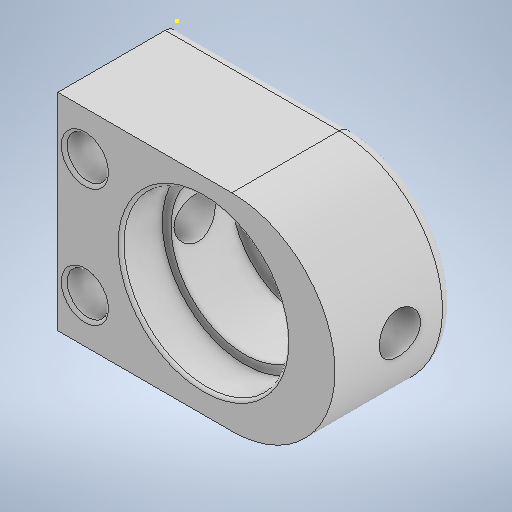
# Autodesk Inventor part: Rodamiento grande
Saved by Autodesk Inventor 2025 (Build 290162000, 162)
## iProperties
Created: 2025-05-21
Part Number: Rodamiento grande
Material: Genérico
Document SubType Name: Modeling
Designer: STEVEN LONDOÑO
Density: 1 g/cm^3
Appearance: Valor por defecto
Author: STEVEN LONDOÑO
Autodesk Inventor part; units mm, degrees
ref_plane "YZ Plane" through (0, 0, 0) normal (1, 0, 0) x (0, 1, 0)
ref_plane "XZ Plane" through (0, 0, 0) normal (0, 1, 0) x (-1, 0, 0)
sketch "Boceto1" plane through (0, 0, 0) normal (0, 0, 1) x (1, 0, 0)
  line L0 (42.7171, -0.3462) -> (13.2171, -0.3462)
  circle A0 centre (37.9098, -17.5) radius 13.97
  line L1 (13.2171, -0.3462) -> (13.2171, -35.3462)
  line L2 (13.2171, -0.3462) -> (13.2171, -35.3462)
  line L3 (13.2171, -35.3462) -> (42.7171, -35.3462)
  arc A1 (42.7171, -35.3462) -> (42.7171, -0.3462) centre (42.7171, -17.8462) ccw
  circle A2 centre (37.9098, -17.5) radius 6
  circle A3 centre (37.9098, -17.5) radius 12.5
  circle A4 centre (29.4098, -17.5) radius 1.5
  circle A5 centre (46.4098, -17.5) radius 1.5
  line L4 (22.4098, -0.3462) -> (22.4098, -35.3462)
  line L5 (22.4098, -0.3462) -> (13.2171, -0.3462)
  circle A6 centre (17.8135, -7.8462) radius 2
  circle A7 centre (17.8135, -27.8462) radius 2
  circle A8 centre (17.8135, -7.8462) radius 3.5
  circle A9 centre (17.8135, -27.8462) radius 3.5
  point P0 (0, 0)
  point P1 (38.7171, -2.3462)
  point P2 (38.7171, -33.3462)
  dimension "d4" = 2
  dimension "d5" = 27.94
  dimension "d7" = 33
  dimension "d10" = 12
  dimension "d11" = 25
  dimension "d27" = 4
  dimension "d28" = 4
  dimension "d30" = 20
  dimension "d31" = 7.5
  dimension "d32" = 7
  dimension "d33" = 7
  constraints: 12 end point, 10 centre point, 4 coincident, 2 point on circle, 2 point on line, 1 horizontal, 1 perpendicular, 1 tangent
  measures "d4" distance from line of L0 point (38.717, -2.346)
  measures "d5" diameter of A0
  measures "d7" distance from line of L0 point (38.717, -33.346)
  measures "d10" diameter of A2
  measures "d11" diameter of A3
  measures "d27" diameter of A6
  measures "d28" diameter of A7
  measures "d30" distance of A7.centre A6.centre
  measures "d31" distance from line of L0 A6.centre
  measures "d32" diameter of A8
  measures "d33" diameter of A9
extrude "Extrusión1" add sketch "Boceto1" along normal blind 20.2 contours A1 L3 L4 L0
extrude "Extrusión2" add sketch "Boceto1" along normal blind 20.2 contours L4 L3 L1 L0
extrude "Extrusión3" add sketch "Boceto1" along normal blind 9 contours A8 | A9
extrude "Extrusión4" add sketch "Boceto1" along normal blind 13.2 contours A0
extrude "Extrusión5" add sketch "Boceto1" along normal blind 3 contours A3
sketch "Boceto2" plane through (13.2171, -35.3462, 0) normal (-1, 0, 0) x (0, 0, 1)
  point P0 (0, 35.3462)
ref_plane "Plano de trabajo1" through (60.2171, -17.8462, 0) normal (-1, 0, 0) x (0, 0, 1)
sketch "Boceto3" plane through (60.2171, -17.8462, 0) normal (-1, 0, 0) x (0, 0, 1)
  line L0 (20.2, -17.5) -> (20.2, 17.5) projected
  line L1 (20.2, 0) -> (9.2, 0)
  circle A0 centre (9.2, 0) radius 3.5
  point P0 (0, 17.8462)
  dimension "d44" = 11
  dimension "d45" = 7
  constraints: 2 end point, 1 centre point, 1 coincident, 1 horizontal, 1 midpoint
  measures "d44" distance of L1.start L1.end
  measures "d45" diameter of A0
hole "Agujero1" at (60.2171, -17.8462, 9.2) direction (-1, 0, 0) diameter 7 end through all
fillet "Empalme1" radius 2 3 edges at (27.9671, -0.3462, 0) (27.9671, -35.3462, 0) (60.2171, -17.8462, 0)
fillet "Empalme2" radius 0.5 1 edges at (31.9098, -17.5, 0)
fillet "Empalme3" radius 0.5 1 edges at (23.9398, -17.5, 20.2)
fillet "Empalme4" radius 0.5 1 edges at (14.3135, -7.8462, 20.2)
fillet "Empalme5" radius 0.5 1 edges at (14.3135, -27.8462, 20.2)
